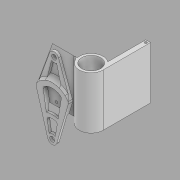
# Autodesk Inventor part: top_frame
Saved by Autodesk Inventor 2020 (Build 240168000, 168)
## iProperties
Created: 2020-03-09
Part Number: top_frame
Material: Generic
Document SubType Name: Modeling
Designer: xXxMrMayhemxXx
Density: 1 g/cm^3
Appearance: Default
Author: xXxMrMayhemxXx
Autodesk Inventor part; units mm, degrees
ref_plane "XZ Plane" through (0, 0, 0) normal (0, 1, 0) x (-1, 0, 0)
sketch "Sketch1" plane through (0, 0, 0) normal (0, 1, 0) x (-1, 0, 0)
  circle A0 centre (0, 0) radius 2
  circle A1 centre (0, 0) radius 2.5
  dimension "d0" = 4
  dimension "d1" = 5
  constraints: 2 centre point, 2 coincident
  measures "d0" diameter of A0
  measures "d1" diameter of A1
extrude "Extrusion1" add sketch "Sketch1" against normal blind 8
ref_plane "Work Plane2" through (0, 0, 0.5) normal (0, 0, 1) x (1, 0, 0)
sketch "Sketch3" plane through (0, 0, 0.5) normal (0, 0, 1) x (1, 0, 0)
  line L0 (-2.5, -8) -> (2.5, -8) projected
  line L1 (-2.5, 0) -> (-9.5, 0)
  line L2 (-10.5, -1) -> (-10.5, -7)
  line L3 (-9.5, -8) -> (-2.5, -8)
  line L4 (-2.5, -8) -> (-2.25, -8)
  line L5 (-2.25, -8) -> (-2.25, 0)
  line L6 (2.5, 0) -> (-2.5, 0) projected
  line L7 (-2.25, 0) -> (-2.5, 0)
  line L8 (-9.5, -8) -> (-10.5, -8)
  line L9 (-10.5, -8) -> (-10.5, -7)
  line L10 (-9.5, 0) -> (-10.5, 0)
  line L11 (-10.5, -1) -> (-10.5, 0)
  point P0 (0, 0)
  point P1 (-9.5, -1)
  dimension "d6" = 8
  dimension "d8" = 0.25
  constraints: 20 end point, 3 point on line, 2 collinear, 2 horizontal, 2 parallel, 2 perpendicular
  measures "d6" distance of L1.start L10.end
  measures "d8" distance of L3.end L4.end
extrude "Extrusion2" add sketch "Sketch3" against normal blind 0.5
sketch "Sketch13" plane through (0, 0, 0.5) normal (0, 0, 1) x (1, 0, 0)
  circle A0 centre (-6.8, -7.25) radius 0.25
  line L0 (-2.4495, 0) -> (-2.4495, -8) projected
  line L1 (-2.4495, 0) -> (-10.5, 0) projected
  line L2 (-10.5, 0) -> (-10.5, -8) projected
  line L3 (-10.5, -8) -> (-2.4495, -8) projected
  point P0 (0, 0)
  dimension "d77" = 0.5
  dimension "d78" = 3.7
  dimension "d79" = 0.75
  constraints: 1 centre point
  measures "d77" diameter of A0
  measures "d78" distance from line of L2 A0.centre
  measures "d79" distance from line of L3 A0.centre
extrude "Extrusion12" cut sketch "Sketch13" against normal through all contours A0
ref_plane "Work Plane3" through (2, 0, 0) normal (1, 0, 0) x (0, 1, 0)
sketch "Sketch16" plane through (2, 0, 0) normal (1, 0, 0) x (0, 1, 0)
  line L0 (-8, 0) -> (-8, 0.5) projected
  line L1 (-8, 0) -> (-8, -10)
  line L2 (-8, -10) -> (0, -10)
  line L3 (0, -10) -> (0, 0)
  line L4 (-8, 0) -> (0, 0) projected
  dimension "d63" = 10
  constraints: 6 end point, 2 parallel, 2 perpendicular
  measures "d63" distance between parallel lines of L2 L4
extrude "Extrusion15" add sketch "Sketch16" along normal mid plane 1
sketch "Sketch17" plane through (0, 0, 0) normal (0, 1, 0) x (1, 0, 0)
  circle A0 centre (0, 0) radius 2
  circle A1 centre (0, 0) radius 2.5
  line L0 (1.5, 0) -> (1.5, 1.3229) projected
  line L1 (2, 0) -> (1.5, 0) projected
  line L2 (2.5, 10) -> (2.5, 0) projected
  dimension "d67" = 5
  dimension "d66" = 4
  constraints: 2 coincident, 1 centre point, 1 horizontal alignment, 1 other
  measures "d66" diameter of A0
extrude "Extrusion16" cut sketch "Sketch17" against normal through all contours L1 L0 A0 picked at (1.5908, 0.7499)
sketch "Sketch18" plane through (0, -8, 0) normal (0, -1, 0) x (1, 0, 0)
  line L0 (1.5, -10) -> (2.5, -10) projected
  line L1 (2.5, 0) -> (2.5, -10) projected
  line L2 (1.5, -10) -> (1.5, -2) projected
  line L3 (1.5, -9.5) -> (2.5, -9.5)
  line L4 (2, -10) -> (2, -9.5)
  circle A0 centre (2, -9.5) radius 0.25
  point P0 (0, 0)
  dimension "d70" = 0.5
  dimension "d71" = 0.5
  constraints: 4 end point, 2 midpoint, 2 point on line, 1 centre point, 1 coincident, 1 horizontal, 1 parallel
  measures "d70" diameter of A0
  measures "d71" distance of L4.start L4.end
extrude "Extrusion17" cut sketch "Sketch18" against normal through all contours A0 L3 L4 | L4 L3 A0 | A0 L3
sketch "Sketch19" plane through (0, 0, 0) normal (0, 1, 0) x (1, 0, 0)
  circle A0 centre (2, 9.5) radius 0.25 projected
  circle A1 centre (0, 0) radius 2 projected
  arc A2 (1.5, 2) -> (-2.5, 0) centre (0, 0) ccw projected
  line L0 (-10.5, 0) -> (-2.5, 0) projected
  line L1 (-10.5, -0.5) -> (-10.5, 0) projected
  line L2 (-2.4495, -0.5) -> (-10.5, -0.5) projected
  arc A3 (-2.4495, -0.5) -> (2.5, 0) centre (0, 0) ccw projected
  line L3 (2.5, 10) -> (2.5, 0) projected
  line L4 (1.5, 10) -> (2.5, 10) projected
  line L5 (1.5, 2) -> (1.5, 10) projected
extrude "Extrusion18" add sketch "Sketch19" along normal blind 3
sketch "Sketch20" plane through (0, 0, 0.5) normal (0, 0, 1) x (1, 0, 0)
  circle A0 centre (-6.8, -7.25) radius 0.25 projected
  circle A1 centre (-6.8, -7.25) radius 0.25 projected
  circle A2 centre (-6.8, 1.199) radius 0.5
  point P0 (0, 0)
  dimension "d82" = 1
  dimension "d83" = 8.449
  constraints: 1 centre point
  measures "d82" diameter of A2
  measures "d83" distance of A2.centre A0.centre
extrude "Extrusion19" cut sketch "Sketch20" against normal through all contours A2
sketch "Sketch21" plane through (0, 0, 0.5) normal (0, 0, 1) x (1, 0, 0)
  circle A0 centre (-6.8, -7.25) radius 0.25 projected
  circle A1 centre (-6.8, 1.199) radius 0.5 projected
  circle A2 centre (-6.8, -7.25) radius 0.25 projected
  line L0 (-2.4495, 3) -> (-2.4495, -8) projected
  line L1 (-10.5, 3) -> (-2.4495, 3) projected
  line L2 (-10.5, 3) -> (-10.5, -8) projected
  line L3 (-10.5, -8) -> (-2.4495, -8) projected
  line L4 (-6.8, -7.25) -> (-9.8, -7.25)
  line L5 (-6.8, -7.25) -> (-3.8, -7.25)
  arc A3 (-3.8, -7.25) -> (-9.8, -7.25) centre (-6.8, -7.25) ccw
  arc A4 (-3.3359, -5.25) -> (-10.2641, -5.25) centre (-6.8, -7.25) ccw
  line L6 (-6.8, -7.25) -> (-3.3359, -5.25)
  line L7 (-6.8, -7.25) -> (-10.2641, -5.25)
  point P0 (0, 0)
  point P1 (-9.3981, -5.75)
  point P2 (-4.2019, -5.75)
  dimension "d86" = 3
  dimension "d87" = 3
  dimension "d92" = 3
  dimension "d93" = 1
  dimension "d94" = 30
  dimension "d95" = 30
  constraints: 8 end point, 4 point on circle, 2 centre point, 1 horizontal, 1 point on line
  measures "d86" distance of L4.start L4.end
  measures "d87" distance of L4.start L5.end
  measures "d92" radius of A3
  measures "d93" radial gap between concentric circles of A3 A4
  measures "d94" angle of L5 L6
  measures "d95" angle of L7 L4
ref_plane "Work Plane4" through (0, 0, 0.9) normal (0, 0, 1) x (1, 0, 0)
sketch "Sketch22" plane through (0, 0, 0.9) normal (0, 0, 1) x (1, 0, 0)
  arc A0 (-3.3359, -5.25) -> (-10.2641, -5.25) centre (-6.8, -7.25) ccw projected
  arc A1 (-3.8, -7.25) -> (-9.8, -7.25) centre (-6.8, -7.25) ccw projected
  line L0 (-6.8, -7.25) -> (-3.3359, -5.25) projected
  line L1 (-6.8, -7.25) -> (-10.2641, -5.25) projected
  circle A2 centre (-6.8, -7.25) radius 0.25 projected
  circle A3 centre (-6.8, -7.25) radius 0.25 projected
  line L2 (-6.8, -7.25) -> (-6.8, -13.551)
  circle A4 centre (-6.8, -13.551) radius 0.5
  circle A5 centre (-6.8, -13.551) radius 1
  line L3 (-6.8, -13.551) -> (-5.8, -13.551)
  line L4 (-6.8, -13.551) -> (-7.8, -13.551)
  line L5 (-6.8, -13.551) -> (-6.1572, -12.785)
  line L6 (-6.8, -13.551) -> (-7.4428, -12.785)
  line L7 (-6.1572, -12.785) -> (-4.8455, -4.9741)
  line L8 (-7.4428, -12.785) -> (-8.7545, -4.9741)
  line L9 (-3.3359, -5.25) -> (-5.84, -13.8311)
  line L10 (-9.778, -6.8875) -> (-7.7603, -13.8301)
  arc A6 (-5.6868, -9.9837) -> (-7.9132, -9.9837) centre (-6.8, -13.551) ccw
  arc A7 (-5.5616, -9.2383) -> (-8.0384, -9.2383) centre (-6.8, -13.551) ccw
  line L11 (-9.778, -6.8875) -> (-10.2641, -5.25)
  point P0 (0, 0)
  dimension "d97" = 1
  dimension "d98" = 6.301
  dimension "d99" = 2
  dimension "d100" = 50
  dimension "d101" = 50
  constraints: 20 end point, 13 point on circle, 5 point on line, 4 centre point, 2 coincident, 2 tangent, 1 perpendicular, 1 vertical
  measures "d97" diameter of A4
  measures "d98" distance of L2.start L2.end
  measures "d99" diameter of A5
  measures "d100" angle of L3 L5
  measures "d101" angle of L6 L4
extrude "Extrusion21" add sketch "Sketch22" along normal blind 0.5 contours L0 A1 L1 A0 | L9 A1 L0 | L1 A1 L11 | L0 L7 A1 | A1 L9 A5 L7 L0 | L1 L8 A5 L10 A1 | A1 L8 L1 | A5 L4 A4 L3 | L7 A6 L2 A7 | L3 A4 L5 A5 | A7 L2 A6 L8 | A5 L6 A4 L4 | L5 A4 L2 A5 | A5 L2 A4 L6
extrude "Extrusion22" add sketch "Sketch21" along normal up to surface (0.4 mm away) contours A3 L7 A4 L6
sketch "Sketch23" plane through (0, 0, 0.5) normal (0, 0, 1) x (1, 0, 0)
  line L0 (-5.84, -13.8311) -> (-3.3359, -5.25) projected
  line L1 (-4.8455, -4.9741) -> (-5.5616, -9.2383) projected
  line L2 (-8.0384, -9.2383) -> (-8.7545, -4.9741) projected
  line L3 (-10.2641, -5.25) -> (-9.778, -6.8875) projected
  line L4 (-9.778, -6.8875) -> (-7.7603, -13.8301) projected
  line L5 (-10.5, -8) -> (-2.4495, -8) projected
  arc A0 (-4.2019, -5.75) -> (-9.3981, -5.75) centre (-6.8, -7.25) ccw projected
  line L6 (-3.3359, -5.25) -> (-4.2019, -5.75) projected
  line L7 (-9.3981, -5.75) -> (-10.2641, -5.25) projected
  point P0 (0, 0)
  point P1 (-5.3536, -8)
  point P2 (-4.1384, -8)
  point P3 (-9.4547, -8)
  point P4 (-8.2464, -8)
extrude "Extrusion23" add sketch "Sketch23" along normal up to surface (0.4 mm away) contours L5 L1 A0 L6 L0 | L5 L4 L3 L7 A0 L2
fillet "Fillet1" radius 0.5 2 edges at (-4.8455, -4.9741, 0.95) (-8.7545, -4.9741, 0.95)
fillet "Fillet2" radius 0.4 2 edges at (-8.8505, -8, 0.9) (-4.746, -8, 0.9)
fillet "Fillet3" radius 0.5 4 edges at (-5.6868, -9.9837, 1.15) (-7.9132, -9.9837, 1.15) (-3.3359, -5.25, 0.95) (-10.2641, -5.25, 0.95)
sketch "Sketch24" plane through (0, 0, 0.5) normal (0, 0, 1) x (1, 0, 0)
  line L0 (-3.3981, -5.4633) -> (-4.1384, -8) projected
  line L1 (-4.1384, -8) -> (-2.4495, -8) projected
  line L2 (-2.4495, 3) -> (-2.4495, -8) projected
  line L3 (-10.5, 3) -> (-2.4495, 3) projected
  line L4 (-10.5, 3) -> (-10.5, -8) projected
  line L5 (-10.5, -8) -> (-9.4547, -8) projected
  line L6 (-9.4547, -8) -> (-9.778, -6.8875) projected
  line L7 (-9.778, -6.8875) -> (-10.2005, -5.4644) projected
  arc A0 (-10.1385, -5.0467) -> (-10.2005, -5.4644) centre (-9.7211, -5.3221) ccw projected
  arc A1 (-3.4607, -5.0479) -> (-10.1385, -5.0467) centre (-6.8, -7.25) ccw projected
  arc A2 (-3.3981, -5.4633) -> (-3.4607, -5.0479) centre (-3.8781, -5.3232) ccw projected
  circle A3 centre (-6.8, 1.199) radius 0.5 projected
  line L8 (-9.4547, -8) -> (-9.778, -6.8875) projected
  line L9 (-9.4547, -8) -> (-10.5, -4.8819)
  line L10 (-10.5, 3) -> (-10.5, -8) projected
  line L11 (-10.5, -4.8819) -> (-7.6312, 3)
  point P0 (0, 0)
  dimension "d119" = 2
  dimension "d120" = 20
  constraints: 4 end point, 2 point on line
  measures "d119" angle of L9 L7
  measures "d120" angle of L4 L11
extrude "Extrusion24" cut sketch "Sketch24" against normal blind 0.5 contours L11 L4 L3 | L9 L5 L4
chamfer "Chamfer2" distance 0.5 angle 45 3 edges at (-5.0656, 3, 0) (-9.0656, -0.941, 0) (-9.9773, -6.441, 0)
fillet "Fillet4" radius 1 2 edges at (-2.4495, -2.5, 0.5) (-2.5, -2.75, 0)
sketch "Sketch26" plane through (0, 0, 0.5) normal (0, 0, 1) x (1, 0, 0)
  arc A0 (-3.4607, -5.0479) -> (-10.1385, -5.0467) centre (-6.8, -7.25) ccw projected
  arc A1 (-10.1385, -5.0467) -> (-10.2005, -5.4644) centre (-9.7211, -5.3221) ccw projected
  arc A2 (-3.3981, -5.4633) -> (-3.4607, -5.0479) centre (-3.8781, -5.3232) ccw projected
  line L0 (-5.84, -13.8311) -> (-3.3981, -5.4633) projected
  line L1 (-10.2005, -5.4644) -> (-9.778, -6.8875) projected
  circle A3 centre (-6.8, 1.199) radius 0.5 projected
  circle A4 centre (-6.8, 1.199) radius 1
  arc A5 (-3.3981, -5.4633) -> (-3.4607, -5.0479) centre (-3.8781, -5.3232) ccw projected
  line L2 (-3.3837, -5.2487) -> (-5.8605, 1.5417)
  line L3 (-10.2157, -5.2486) -> (-7.7395, 1.5416)
  arc A6 (-4.8951, -5.2696) -> (-5.1058, -4.7742) centre (-5.3882, -5.1868) ccw projected
  arc A7 (-8.4942, -4.7742) -> (-8.7049, -5.2696) centre (-8.2118, -5.1868) ccw projected
  line L4 (-4.9281, -4.9911) -> (-6.2648, 0.3543)
  line L5 (-8.6719, -4.9911) -> (-7.3356, 0.3545)
  point P0 (0, 0)
  point P1 (-5.2894, -3.5462)
  point P2 (-3.4519, -5.0619)
  point P3 (-10.1469, -5.0599)
  point P4 (-8.3107, -3.5463)
  dimension "d127" = 2
  dimension "d128" = 6
  dimension "d129" = 6
  constraints: 9 point on circle, 8 end point, 2 tangent, 1 centre point, 1 coincident
  measures "d127" diameter of A4
  measures "d128" angle of L4 L2
  measures "d129" angle of L3 L5
extrude "Extrusion25" add sketch "Sketch26" along normal blind 0.5 contours A0 L4 A4 L2 A2 | A0 A1 L3 A4 L5 | A4
chamfer "Chamfer3" distance 0.399 angle 45 4 edges at (-4.2615, -4.1588, 1) (-3.4562, -5.0549, 1) (-9.338, -4.1583, 1) (-10.1427, -5.0532, 1)
chamfer "Chamfer4" distance 0.89 angle 45 1 edges at (-6.8001, -3.25, 0.5)
body "Solid1"
